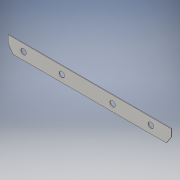
# Autodesk Inventor part: OutsidePlate2
Saved by Autodesk Inventor 2016 (Build 200138000, 138)
## iProperties
Created: 2017-01-21
Part Number: OutsidePlate2
Material: Generic
Document SubType Name: Modeling
Designer: hamblettk
Density: 1 g/cm^3
Appearance: Default
Author: hamblettk
Autodesk Inventor part; units mm, degrees
ref_plane "YZ Plane" through (0, 0, 0) normal (1, 0, 0) x (0, 1, 0)
ref_plane "XZ Plane" through (0, 0, 0) normal (0, 1, 0) x (-1, 0, 0)
ref_plane "XY Plane" through (0, 0, 0) normal (0, 0, 1) x (1, 0, 0)
sketch "Sketch1" plane through (0, 0, 0) normal (0, 0, 1) x (1, 0, 0)
  line L0 (0, 0) -> (850.9, 0)
  line L1 (850.9, 0) -> (850.9, 76.2)
  line L2 (850.9, 76.2) -> (0, 76.2)
  line L3 (0, 76.2) -> (0, 0)
  dimension "d0" = 850.9
  dimension "d1" = 76.2
  constraints: 8 end point, 2 parallel, 1 horizontal, 1 perpendicular
  measures "d0" distance of L2.end L1.end
  measures "d1" distance of L1.end L0.end
extrude "Extrusion1" add sketch "Sketch1" along normal blind 3.175
sketch "Sketch2" plane through (0, 0, 3.175) normal (0, 0, 1) x (1, 0, 0)
  line L0 (0, 0) -> (25.4, 0)
  line L1 (0, 0) -> (0, 38.1)
  line L2 (0, 38.1) -> (25.4, 0)
  line L3 (0, 0) -> (850.9, 0) projected
  line L4 (850.9, 0) -> (850.9, 38.1)
  line L5 (850.9, 0) -> (850.9, 76.2) projected
  line L6 (850.9, 0) -> (825.5, 0)
  line L7 (825.5, 0) -> (850.9, 38.1)
  line L8 (0, 38.1) -> (0, 36.5125)
  line L9 (0, 36.5125) -> (0, 39.6875)
  circle A0 centre (280.2509, 36.5125) radius 14.2875
  circle A1 centre (545.2491, 36.5125) radius 14.2875
  circle A2 centre (80.2257, 39.6875) radius 14.2875
  circle A3 centre (745.2743, 39.6875) radius 14.2875
  dimension "d4" = 25.4
  dimension "d5" = 38.1
  dimension "d6" = 38.1
  dimension "d7" = 25.4
  dimension "d13" = 28.575
  dimension "d14" = 28.575
  dimension "d17" = 28.575
  dimension "d19" = 28.575
  constraints: 16 end point, 4 centre point, 1 horizontal, 1 midpoint, 1 point on line
  measures "d4" distance of L0.start L0.end
  measures "d5" distance of L0.start L1.end
  measures "d6" distance of L3.end L4.end
  measures "d7" distance of L3.end L6.end
  measures "d13" diameter of A0
  measures "d14" diameter of A1
  measures "d17" diameter of A2
  measures "d19" diameter of A3
extrude "Extrusion2" cut sketch "Sketch2" against normal blind 3.175
body "Solid1"
